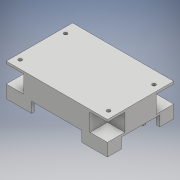
# Autodesk Inventor part: cmoda7
Saved by Autodesk Inventor 2018 (Build 220112000, 112)
## iProperties
Created: 2019-07-22
Part Number: cmoda7
Material: 一般
Document SubType Name: Modeling
Designer: guest1
Density: 1 g/cm^3
Appearance: 既定
Author: guest1
Autodesk Inventor part; units mm, degrees
ref_plane "YZ Plane" through (0, 0, 0) normal (1, 0, 0) x (0, 1, 0)
ref_plane "XZ Plane" through (0, 0, 0) normal (0, 1, 0) x (-1, 0, 0)
ref_plane "XY Plane" through (0, 0, 0) normal (0, 0, 1) x (1, 0, 0)
sketch "スケッチ3" plane through (0, 0, 0) normal (0, 0, 1) x (1, 0, 0)
  line L0 (43.5, -28.5) -> (-43.5, -28.5)
  line L1 (-43.5, -28.5) -> (-43.5, 28.5)
  line L2 (-43.5, 28.5) -> (43.5, 28.5)
  line L3 (43.5, 28.5) -> (43.5, -28.5)
  line L4 (43.5, -28.5) -> (-43.5, 28.5) construction
  line L5 (-43.5, -28.5) -> (43.5, 28.5) construction
  point P0 (0, 0)
  dimension "d4" = 57
  dimension "d5" = 87
  constraints: 12 end point, 2 midpoint, 2 parallel, 1 horizontal, 1 perpendicular
  measures "d4" distance of L2.end L0.start
  measures "d5" distance of L1.end L2.end
extrude "枠" add sketch "スケッチ3" along normal blind 70
sketch "スケッチ4" plane through (0, 0, 0) normal (0, 0, -1) x (-1, 0, 0)
  line L0 (40.6, -26.5) -> (-40.6, -26.5)
  line L1 (-40.6, -26.5) -> (-40.6, 26.5)
  line L2 (-40.6, 26.5) -> (40.6, 26.5)
  line L3 (40.6, 26.5) -> (40.6, -26.5)
  line L4 (40.6, -26.5) -> (-40.6, 26.5) construction
  line L5 (-40.6, -26.5) -> (40.6, 26.5) construction
  point P0 (0, 0)
  dimension "d8" = 81.2
  dimension "d9" = 53
  constraints: 12 end point, 2 midpoint, 2 parallel, 1 horizontal, 1 perpendicular
  measures "d8" distance of L1.end L2.end
  measures "d9" distance of L0.end L1.end
extrude "本体" cut sketch "スケッチ4" against normal blind 56
sketch "スケッチ5" plane through (-43.5, 28.5, 0) normal (0, 1, 0) x (1, 0, 0)
  line L0 (0, 0) -> (0, -70) projected
  line L1 (87, 0) -> (87, -70) projected
  line L2 (0, -51) -> (87, -51)
  line L3 (87, -51) -> (87, -55)
  line L4 (87, -55) -> (0, -55)
  line L5 (0, -55) -> (0, -51)
  line L6 (87, -70) -> (0, -70) projected
  point P0 (43.5, 0)
  dimension "d12" = 15
  dimension "d13" = 4
  constraints: 8 end point, 2 parallel, 2 point on line, 1 horizontal, 1 perpendicular
  measures "d12" distance between parallel lines of L6 L4
  measures "d13" distance between parallel lines of L4 L2
extrude "台" add sketch "スケッチ5" against normal blind 55 contours L2 L1 L4 L0
sketch "スケッチ6" plane through (0, 0, 0) normal (0, 0, -1) x (-1, 0, 0)
  line L0 (40.6, -26.5) -> (40.6, 26.5) projected
  line L1 (43.1, 19.5) -> (40.6, 19.5)
  line L2 (40.6, 19.5) -> (40.6, 13.5)
  line L3 (40.6, 13.5) -> (43.1, 13.5)
  line L4 (43.1, 13.5) -> (43.1, 19.5)
  line L5 (40.6, 26.5) -> (-40.6, 26.5) projected
  line L6 (32.6, 26.5) -> (26.6, 26.5)
  line L7 (26.6, 26.5) -> (26.6, 28)
  line L8 (26.6, 28) -> (32.6, 28)
  line L9 (32.6, 28) -> (32.6, 26.5)
  line L10 (-26.6, 26.5) -> (-32.6, 26.5)
  line L11 (-32.6, 26.5) -> (-32.6, 28)
  line L12 (-32.6, 28) -> (-26.6, 28)
  line L13 (-26.6, 28) -> (-26.6, 26.5)
  line L14 (-40.6, -26.5) -> (-40.6, 26.5) projected
  point P0 (0, 0)
  dimension "d16" = 2.5
  dimension "d17" = 13
  dimension "d18" = 6
  dimension "d19" = 1.5
  dimension "d20" = 8
  dimension "d21" = 6
  dimension "d22" = 1.5
  dimension "d23" = 6
  dimension "d24" = 8
  constraints: 24 end point, 6 parallel, 3 horizontal, 3 perpendicular, 3 point on line
  measures "d16" distance of L1.start L1.end
  measures "d17" distance between parallel lines of L5 L3
  measures "d18" distance of L3.end L1.start
  measures "d19" distance of L8.end L6.start
  measures "d20" distance from line of L0.end L9
  measures "d21" distance of L6.start L6.end
  measures "d22" distance between parallel lines of L12 L10
  measures "d23" distance of L11.end L12.end
  measures "d24" distance between parallel lines of L14 L11
extrude "溝" cut sketch "スケッチ6" against normal blind 51
sketch "スケッチ7" plane through (40.6, -26.5, 0) normal (-1, 0, 0) x (0, 0, 1)
  line L0 (51, 10) -> (31, 10)
  line L1 (31, 10) -> (31, 43)
  line L2 (31, 43) -> (51, 43)
  line L3 (51, 43) -> (51, 10)
  line L4 (51, 53) -> (0, 53) projected
  line L5 (51, 0) -> (51, 53) projected
  point P0 (0, 26.5)
  point P1 (0, 0)
  dimension "d27" = 10
  dimension "d28" = 10
  dimension "d29" = 20
  dimension "d30" = 0
  constraints: 8 end point, 2 parallel, 1 horizontal, 1 perpendicular
  measures "d27" distance from line of point (0, 0) L0
  measures "d28" distance between parallel lines of L4 L2
  measures "d29" distance between parallel lines of L3 L1
  measures "d30" distance between parallel lines of L5 L3
extrude "USB穴" cut sketch "スケッチ7" along normal through all both and the other way through all
sketch "スケッチ8" plane through (-26.6, 26.5, 0) normal (0, -1, 0) x (1, 0, 0)
  line L0 (67.2, 51) -> (-14, 51) projected
  line L1 (48.2, 31) -> (5, 31)
  line L2 (5, 31) -> (5, 51)
  line L3 (5, 51) -> (48.2, 51)
  line L4 (48.2, 51) -> (48.2, 31)
  line L5 (53.2, 0) -> (53.2, 51) projected
  line L6 (0, 51) -> (0, 0) projected
  point P0 (26.6, 0)
  dimension "d33" = 5
  dimension "d34" = 5
  dimension "d35" = 20
  constraints: 8 end point, 2 parallel, 1 horizontal, 1 perpendicular, 1 point on line
  measures "d33" distance between parallel lines of L5 L4
  measures "d34" distance between parallel lines of L6 L2
  measures "d35" distance between parallel lines of L0 L1
extrude "ボタン押下用穴" cut sketch "スケッチ8" along normal through all both and the other way through all
sketch "su" plane through (-32.6, 26.5, 51) normal (0, 0, -1) x (-1, 0, 0)
  line L0 (-64.2, -53) -> (-61.7, -53)
  line L1 (-61.7, -53) -> (-61.7, -52)
  line L2 (-61.7, -52) -> (-64.2, -52)
  line L3 (-64.2, -52) -> (-64.2, -53)
  line L4 (-3.5, -53) -> (-1, -53)
  line L5 (-1, -53) -> (-1, -52)
  line L6 (-1, -52) -> (-3.5, -52)
  line L7 (-3.5, -52) -> (-3.5, -53)
  line L8 (-74.2, -22.5) -> (-73.2, -22.5)
  line L9 (-73.2, -22.5) -> (-73.2, -20)
  line L10 (-73.2, -20) -> (-74.2, -20)
  line L11 (-74.2, -20) -> (-74.2, -22.5)
  line L12 (-73.2, -53) -> (-73.2, -43) projected
  line L13 (8, -53) -> (-73.2, -53) projected
  line L14 (8, -13) -> (8, -53) projected
  point P0 (-32.6, -26.5)
  point P1 (-65.2, 0)
  point P2 (8, -40)
  dimension "d49" = 9
  dimension "d50" = 0
  dimension "d51" = 2.5
  dimension "d52" = 1
  dimension "d53" = 20
  dimension "d54" = 1
  dimension "d56" = 2.5
  dimension "d57" = 9
  dimension "d58" = 1
  dimension "d59" = 2.5
  dimension "d60" = 0
  constraints: 24 end point, 6 parallel, 3 horizontal, 3 perpendicular
  measures "d49" distance between parallel lines of L12 L3
  measures "d50" distance between parallel lines of L13 L0
  measures "d51" distance of L1.end L2.end
  measures "d52" distance of L0.end L1.end
  measures "d53" distance from line of point (-65.2, 0) L10
  measures "d54" distance of L8.start L8.end
  measures "d56" distance of L9.end L8.end
  measures "d57" distance between parallel lines of L14 L5
  measures "d58" distance of L6.end L4.start
  measures "d59" distance of L5.end L6.end
  measures "d60" distance between parallel lines of L13 L4
extrude "凸" add sketch "su" along normal blind 3
sketch "スケッチ11" plane through (0, 0, 70) normal (0, 0, 1) x (1, 0, 0)
  line L0 (43.5, -28.5) -> (-43.5, -28.5) projected
  line L1 (43.5, 28.5) -> (-43.5, 28.5) projected
  line L2 (-43.5, -28.5) -> (43.5, -28.5)
  line L3 (43.5, -28.5) -> (43.5, 28.5)
  line L4 (43.5, 28.5) -> (-43.5, 28.5)
  line L5 (-43.5, 28.5) -> (-43.5, -28.5)
  point P0 (0, 0)
  constraints: 8 end point, 2 parallel, 1 horizontal, 1 perpendicular
extrude "底面" add sketch "スケッチ11" against normal up to surface (15 mm away)
sketch "スケッチ13" plane through (-43.5, -28.5, 0) normal (0, -1, 0) x (1, 0, 0)
  line L0 (87, 0) -> (87, 70) projected
  line L1 (87, 53) -> (72, 53)
  line L2 (72, 53) -> (72, 68)
  line L3 (72, 68) -> (87, 68)
  line L4 (87, 68) -> (87, 53)
  line L5 (0, 0) -> (0, 70) projected
  line L6 (0, 53) -> (15, 53)
  line L7 (15, 53) -> (15, 68)
  line L8 (15, 68) -> (0, 68)
  line L9 (0, 68) -> (0, 53)
  line L10 (0, 70) -> (87, 70) projected
  point P0 (43.5, 0)
  dimension "d70" = 2
  dimension "d71" = 15
  dimension "d72" = 15
  dimension "d73" = 15
  constraints: 16 end point, 4 parallel, 4 point on line, 2 horizontal, 2 perpendicular
  measures "d70" distance between parallel lines of L10 L3
  measures "d71" distance of L1.start L1.end
  measures "d72" distance of L6.start L6.end
  measures "d73" distance of L6.end L7.end
extrude "ネジ止め1" cut sketch "スケッチ13" against normal blind 15
sketch "スケッチ14" plane through (-43.5, 28.5, 0) normal (0, 1, 0) x (1, 0, 0)
  line L0 (0, 0) -> (0, -70) projected
  line L1 (0, -53) -> (15, -53)
  line L2 (15, -53) -> (15, -68)
  line L3 (15, -68) -> (0, -68)
  line L4 (0, -68) -> (0, -53)
  line L5 (87, 0) -> (87, -53) projected
  line L6 (87, -53) -> (72, -53)
  line L7 (72, -53) -> (72, -68)
  line L8 (72, -68) -> (87, -68)
  line L9 (87, -68) -> (87, -53)
  line L10 (87, -70) -> (0, -70) projected
  point P0 (43.5, 0)
  dimension "d76" = 15
  dimension "d77" = 15
  dimension "d78" = 15
  dimension "d79" = 2
  constraints: 16 end point, 4 parallel, 4 point on line, 2 horizontal, 2 perpendicular
  measures "d76" distance of L1.start L1.end
  measures "d77" distance of L6.start L6.end
  measures "d78" distance of L1.end L2.end
  measures "d79" distance between parallel lines of L10 L3
extrude "ネジ止め2" cut sketch "スケッチ14" against normal blind 15
sketch "スケッチ19" plane through (0, 0, 0) normal (0, 0, -1) x (-1, 0, 0)
  line L0 (-43.5, 28.5) -> (43.5, 28.5) projected
  line L1 (-43.5, -28.5) -> (-28.5, -28.5) projected
  line L2 (43.5, 28.5) -> (-43.5, 28.5)
  line L3 (-43.5, 28.5) -> (-43.5, -28.5)
  line L4 (-43.5, -28.5) -> (43.5, -28.5)
  line L5 (43.5, -28.5) -> (43.5, 28.5)
  point P0 (0, 0)
  constraints: 8 end point, 2 parallel, 1 horizontal, 1 perpendicular
extrude "上面削り" cut sketch "スケッチ19" against normal blind 42
sketch "ネジ穴用" plane through (0, 0, 70) normal (0, 0, 1) x (1, 0, 0)
  line L0 (37.5, 17.5) -> (-38.5, 17.5)
  line L1 (-38.5, 17.5) -> (-38.5, -21.5)
  line L2 (-38.5, -21.5) -> (37.5, -21.5)
  line L3 (37.5, -21.5) -> (37.5, 17.5)
  line L4 (43.5, -28.5) -> (43.5, 28.5) projected
  line L5 (-43.5, -28.5) -> (43.5, -28.5) projected
  point P0 (0, 0)
  dimension "d100" = 39
  dimension "d101" = 76
  dimension "d102" = 6
  dimension "d103" = 7
  constraints: 8 end point, 2 parallel, 1 horizontal, 1 perpendicular
  measures "d100" distance of L2.end L0.start
  measures "d101" distance of L0.start L0.end
  measures "d102" distance between parallel lines of L3 L4
  measures "d103" distance between parallel lines of L5 L2
sketch "スケッチ23" plane through (0, 0, 42) normal (0, 0, -1) x (-1, 0, 0)
  line L0 (-32.6, 26.5) -> (-32.6, 28) projected
  line L1 (-26.6, 28) -> (-26.6, 26.5) projected
  line L2 (-32.6, 28.5) -> (-26.6, 28.5)
  line L3 (-26.6, 28.5) -> (-26.6, 26.5)
  line L4 (-26.6, 26.5) -> (-32.6, 26.5)
  line L5 (-32.6, 26.5) -> (-32.6, 28.5)
  line L6 (26.6, 28) -> (26.6, 26.5) projected
  line L7 (32.6, 26.5) -> (32.6, 28) projected
  line L8 (26.6, 26.5) -> (32.6, 26.5)
  line L9 (32.6, 26.5) -> (32.6, 28.5)
  line L10 (32.6, 28.5) -> (26.6, 28.5)
  line L11 (26.6, 28.5) -> (26.6, 26.5)
  point P0 (0, 0)
  point P1 (26.6, 28.5)
  constraints: 16 end point, 4 parallel, 2 horizontal, 2 perpendicular
extrude "押し出し18" add sketch "スケッチ23" against normal blind 2
hole "穴2" at (-38.5, -21.5, 70) at (37.5, -21.5, 70) at (37.5, 17.5, 70) at (-38.5, 17.5, 70) direction (0, 0, -1) diameter 3 depth 4 tip angle 118
